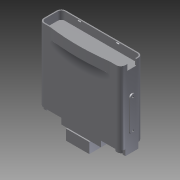
# Autodesk Inventor part: radio
Saved by Autodesk Inventor 2014 (Build 180170000, 170)
## iProperties
Created: 2013-11-09
Part Number: radio
Material: Generic
Document SubType Name: Modeling
Designer: Tyler
Density: 1 g/cm^3
Appearance: Default
Author: Tyler
Autodesk Inventor part; units mm, degrees
ref_plane "YZ Plane" through (0, 0, 0) normal (1, 0, 0) x (0, 1, 0)
ref_plane "XZ Plane" through (0, 0, 0) normal (0, 1, 0) x (-1, 0, 0)
ref_plane "XY Plane" through (0, 0, 0) normal (0, 0, 1) x (1, 0, 0)
sketch "Sketch1" plane through (0, 0, 0) normal (0, 0, 1) x (1, 0, 0)
  line L0 (-62, 19) -> (62, 19)
  line L1 (70, 11) -> (70, -11)
  line L2 (62, -19) -> (-62, -19)
  line L3 (-70, -11) -> (-70, 11)
  arc A0 (-62, 19) -> (-70, 11) centre (-62, 11) ccw
  arc A1 (-70, -11) -> (-62, -19) centre (-62, -11) ccw
  arc A2 (70, 11) -> (62, 19) centre (62, 11) ccw
  arc A3 (62, -19) -> (70, -11) centre (62, -11) ccw
  point P0 (0, 0)
  point P1 (70, -19)
  point P2 (70, 19)
  point P3 (-70, -19)
  dimension "d0" = 140
  dimension "d1" = 38
  dimension "d2" = 70
  dimension "d3" = 19
  dimension "d4" = 8
  dimension "d5" = 8
  dimension "d6" = 8
  dimension "d7" = 8
  constraints: 8 end point, 8 point on circle, 8 tangent, 6 point on line, 4 centre point, 2 parallel, 1 horizontal, 1 perpendicular
  measures "d0" distance of point (70, -19) point (-70, -19)
  measures "d1" distance of point (70, 19) point (70, -19)
  measures "d2" distance from line of L3 point (0, 0)
  measures "d3" distance from line of L2 point (0, 0)
  measures "d4" radius of A0
  measures "d5" radius of A1
  measures "d6" radius of A2
  measures "d7" radius of A3
extrude "Extrusion1" add sketch "Sketch1" against normal blind 18
sketch "Sketch2" plane through (0, 0, 0) normal (0, 0, 1) x (1, 0, 0)
  line L0 (-62, 19) -> (62, 19) projected
  arc A0 (-62, 19) -> (-70, 11) centre (-62, 11) ccw projected
  line L1 (-70, -11) -> (-70, 11) projected
  arc A1 (-70, -11) -> (-62, -19) centre (-62, -11) ccw projected
  line L2 (62, -19) -> (-62, -19) projected
  arc A2 (62, -19) -> (70, -11) centre (62, -11) ccw projected
  line L3 (70, 11) -> (70, -11) projected
  arc A3 (70, 11) -> (62, 19) centre (62, 11) ccw projected
  line L4 (62, 17) -> (-62, 17)
  arc A4 (-62, 17) -> (-68, 11) centre (-62, 11) ccw
  line L5 (-68, 11) -> (-68, -11)
  arc A5 (-68, -11) -> (-62, -17) centre (-62, -11) ccw
  line L6 (-62, -17) -> (62, -17)
  arc A6 (62, -17) -> (68, -11) centre (62, -11) ccw
  line L7 (68, -11) -> (68, 11)
  arc A7 (68, 11) -> (62, 17) centre (62, 11) ccw
  point P0 (0, 0)
  dimension "d10" = 2
  constraints: 8 end point, 8 point on circle, 4 centre point, 7 other
  measures "d10" distance between parallel lines of L4 L0
extrude "Extrusion2" cut sketch "Sketch2" against normal blind 14 contours A7 L7 A6 L6 A5 L5 A4 L4
sketch "Sketch3" plane through (70, -11, 0) normal (1, 0, 0) x (0, 0, -1)
  line L0 (0, 22) -> (0, 0) projected
  line L1 (-6.9158, 18.5) -> (10, 18.5)
  line L2 (10, 18.5) -> (10, 3.5)
  line L3 (10, 3.5) -> (-6.9158, 3.5)
  line L4 (-6.9158, 3.5) -> (-6.9158, 18.5)
  point P0 (0, 11)
  dimension "d13" = 6.9158
  dimension "d14" = 10
  dimension "d15" = 15
  dimension "d16" = 7.5
  constraints: 8 end point, 2 parallel, 1 horizontal, 1 perpendicular
  measures "d13" distance between parallel lines of L4 L0
  measures "d14" distance between parallel lines of L2 L0
  measures "d15" distance of L1.end L2.end
  measures "d16" distance from line of L3 point (0, 11)
extrude "Extrusion3" cut sketch "Sketch3" against normal blind 14
sketch "Sketch4" plane through (0, 0, -14) normal (0, 0, 1) x (1, 0, 0)
  line L0 (-62, -17) -> (62, -17) projected
  line L1 (62, 17) -> (-62, 17) projected
  line L2 (27, 19) -> (32, 19)
  line L3 (32, 19) -> (32, 16)
  line L4 (32, 16) -> (27, 16)
  line L5 (27, 16) -> (27, 19)
  line L6 (32, -19) -> (27, -19)
  line L7 (27, -19) -> (27, -16)
  line L8 (27, -16) -> (32, -16)
  line L9 (32, -16) -> (32, -19)
  line L10 (-42, -19) -> (-47, -19)
  line L11 (-47, -19) -> (-47, -16)
  line L12 (-47, -16) -> (-42, -16)
  line L13 (-42, -16) -> (-42, -19)
  line L14 (70, 7.5) -> (70, -7.5) projected
  line L15 (62, -19) -> (-62, -19) projected
  line L16 (-62, 19) -> (62, 19) projected
  line L17 (-39, 19) -> (-34, 19)
  line L18 (-34, 19) -> (-34, 16)
  line L19 (-34, 16) -> (-39, 16)
  line L20 (-39, 16) -> (-39, 19)
  line L21 (-70, -11) -> (-70, 11) projected
  point P0 (0, 0)
  dimension "d19" = 38
  dimension "d20" = 5
  dimension "d21" = 5
  dimension "d22" = 38
  dimension "d23" = 1
  dimension "d24" = 1
  dimension "d25" = 0
  dimension "d26" = 0
  dimension "d28" = 1
  dimension "d29" = 0
  dimension "d30" = 5
  dimension "d31" = 5
  dimension "d33" = 1
  dimension "d34" = 0
  dimension "d59" = 66
  dimension "d60" = 74
  constraints: 32 end point, 8 parallel, 4 horizontal, 4 perpendicular
  measures "d19" distance from line of L6.start L14
  measures "d20" distance between parallel lines of L9 L7
  measures "d21" distance between parallel lines of L5 L3
  measures "d22" distance between parallel lines of L14 L3
  measures "d23" distance between parallel lines of L4 L1
  measures "d24" distance between parallel lines of L0 L8
  measures "d25" distance between parallel lines of L15 L6
  measures "d26" distance between parallel lines of L16 L2
  measures "d28" distance between parallel lines of L19 L1
  measures "d29" distance between parallel lines of L16 L17
  measures "d30" distance of L18.end L19.end
  measures "d31" distance of L11.end L12.end
  measures "d33" distance between parallel lines of L0 L12
  measures "d34" distance between parallel lines of L15 L10
  measures "d59" distance of L3.end L18.end
  measures "d60" distance between parallel lines of L9 L13
extrude "Extrusion4" add sketch "Sketch4" along normal blind 13 contours L11 L12 L13 L0 | L0 L13 L10 L11 | L7 L8 L9 L0 | L0 L9 L6 L7 | L3 L4 L5 L1 | L1 L5 L2 L3 | L18 L19 L20 L1 | L1 L20 L16 L18
chamfer "Chamfer1" distance 1 distance2 1 1 edges at (-36.5, 16, -1) measured on face at (-36.5, 16, -1.5)
chamfer "Chamfer3" distance 1 distance2 1 1 edges at (29.5, 16, -1) measured on face at (29.5, 16, -1.5)
chamfer "Chamfer4" distance 1 distance2 1 1 edges at (-44.5, -16, -1) measured on face at (-44.5, -16, -1.5)
chamfer "Chamfer5" distance 1 distance2 1 1 edges at (29.5, -16, -1) measured on face at (29.5, -16, -1.5)
sketch "Sketch5" plane through (0, 0, -14) normal (0, 0, 1) x (1, 0, 0)
  line L0 (-39, 17) -> (-62, 17) projected
  arc A0 (-62, 17) -> (-68, 11) centre (-62, 11) ccw projected
  line L1 (-68, 11) -> (-68, -11) projected
  arc A1 (-68, -11) -> (-62, -17) centre (-62, -11) ccw projected
  line L2 (-62, -17) -> (-47, -17) projected
  line L3 (-47, -17) -> (-47, -16) projected
  line L4 (-47, -16) -> (-42, -16) projected
  line L5 (-42, -16) -> (-42, -17) projected
  line L6 (-42, -17) -> (27, -17) projected
  line L7 (27, -17) -> (27, -16) projected
  line L8 (27, -16) -> (32, -16) projected
  line L9 (32, -16) -> (32, -17) projected
  line L10 (32, -17) -> (62, -17) projected
  line L11 (-49, 17) -> (37, 17)
  line L12 (37, 17) -> (37, -17)
  line L13 (37, -17) -> (-49, -17)
  line L14 (-49, -17) -> (-49, 17)
  point P0 (32, 16)
  point P1 (-39, 16)
  point P2 (0, 0)
  dimension "d53" = 10
  dimension "d54" = 5
  constraints: 8 end point, 2 parallel, 2 point on line, 1 horizontal, 1 perpendicular
  measures "d53" distance from line of point (-39, 16) L14
  measures "d54" distance from line of point (32, 16) L12
extrude "Extrusion5" cut sketch "Sketch5" along normal blind 11
sketch "Sketch8" plane through (0, 0, 0) normal (0, 0, 1) x (1, 0, 0)
  line L0 (-70, -11) -> (-70, 11) projected
  line L1 (62, -19) -> (-62, -19) projected
  line L2 (70, -7.5) -> (70, -11) projected
  line L3 (62, -17) -> (-62, -17) projected
  line L4 (0, -22.5) -> (0, -17) construction
  arc A0 (-52, -18.8579) -> (52, -18.8579) centre (0, 350.5357) ccw
  arc A1 (-49.9899, -19.1353) -> (-52, -19) centre (-52, -34) ccw
  arc A2 (52, -19) -> (49.9899, -19.1353) centre (52, -34) ccw
  line L5 (-52, -19) -> (-52, -17)
  line L6 (52, -19) -> (52, -17)
  line L7 (52, -17) -> (-52, -17)
  point P0 (0, 0)
  dimension "d63" = 2
  dimension "d64" = 18
  dimension "d65" = 18
  dimension "d66" = 5.5
  dimension "d67" = 30
  dimension "d68" = 30
  constraints: 9 point on circle, 8 end point, 6 point on line, 4 tangent, 3 centre point, 3 perpendicular, 1 collinear, 1 midpoint
  measures "d63" distance between parallel lines of L1 L3
  measures "d64" distance from line of L2 A2.centre
  measures "d65" distance from line of A1.centre L0
  measures "d66" distance of L4.start L4.end
  measures "d67" diameter of A1
  measures "d68" diameter of A2
extrude "Extrusion8" add sketch "Sketch8" against normal up to surface (18 mm away) contours A0 L1 | L1 A0 L5 L3 L6
sketch "Sketch11" plane through (0, 0, -18) normal (0, 0, -1) x (-1, 0, 0)
  line L0 (62, -19) -> (50.9804, -19) projected
  arc A0 (62, -19) -> (70, -11) centre (62, -11) ccw projected
  line L1 (70, 11) -> (70, -11) projected
  arc A1 (70, 11) -> (62, 19) centre (62, 11) ccw projected
  line L2 (-62, 19) -> (62, 19) projected
  arc A2 (-62, 19) -> (-70, 11) centre (-62, 11) ccw projected
  line L3 (-70, -11) -> (-70, 11) projected
  arc A3 (-70, -11) -> (-62, -19) centre (-62, -11) ccw projected
  line L4 (-50.9804, -19) -> (-62, -19) projected
  line L5 (-50.9804, -19) -> (50.9804, -19)
  point P0 (0, 0)
  constraints: 2 end point, 1 collinear
extrude "Extrusion10" add sketch "Sketch11" along normal blind 107
fillet "Fillet2" radius 60 1 edges at (0, -19, -18)
sketch "Sketch12" plane through (0, 0, -125) normal (0, 0, -1) x (-1, 0, 0)
  line L0 (-62, -19) -> (62, -19) projected
  line L1 (-70, 11) -> (-70, -11) projected
  circle A0 centre (-50, 2) radius 7.5
  point P0 (0, 0)
  dimension "d81" = 15
  dimension "d82" = 21
  dimension "d83" = 20
  constraints: 1 centre point
  measures "d81" diameter of A0
  measures "d82" distance from line of L0 A0.centre
  measures "d83" distance from line of L1 A0.centre
extrude "Extrusion11" add sketch "Sketch12" along normal blind 17
sketch "Sketch13" plane through (0, 0, -125) normal (0, 0, -1) x (-1, 0, 0)
  line L0 (70, -11) -> (70, 11) projected
  line L1 (-70, 11) -> (-70, -11) projected
  line L2 (-70, 11) -> (-65, 11)
  line L3 (-65, 11) -> (-65, -11)
  line L4 (-65, -11) -> (-70, -11)
  line L5 (-70, -11) -> (-70, 11)
  line L6 (70, -11) -> (65, -11)
  line L7 (65, -11) -> (65, 11)
  line L8 (65, 11) -> (70, 11)
  line L9 (70, 11) -> (70, -11)
  point P0 (0, 0)
  dimension "d86" = 0
  dimension "d87" = 0
  dimension "d88" = 0
  dimension "d89" = 5
  dimension "d90" = 0
  dimension "d91" = 0
  dimension "d92" = 0
  dimension "d93" = 5
  constraints: 16 end point, 4 parallel, 2 horizontal, 2 perpendicular
  measures "d86" distance from line of L2 L1.start
  measures "d87" distance from line of L1.end L4
  measures "d88" distance between parallel lines of L1 L5
  measures "d89" distance between parallel lines of L1 L3
  measures "d90" distance between parallel lines of L0 L9
  measures "d91" distance from line of L8 L0.end
  measures "d92" distance from line of L0.start L6
  measures "d93" distance between parallel lines of L9 L7
extrude "Extrusion12" add sketch "Sketch13" along normal blind 10
sketch "Sketch14" plane through (0, 0, -125) normal (0, 0, -1) x (-1, 0, 0)
  line L0 (-62, -19) -> (62, -19) projected
  line L1 (62, 19) -> (-62, 19) projected
  line L2 (-36, 19) -> (32, 19)
  line L3 (32, 19) -> (32, -19)
  line L4 (32, -19) -> (-36, -19)
  line L5 (-36, -19) -> (-36, 19)
  line L6 (70, -11) -> (70, 11) projected
  point P0 (0, 0)
  dimension "d96" = 38
  dimension "d97" = 68
  dimension "d98" = 0
  dimension "d99" = 0
  constraints: 8 end point, 2 parallel, 1 horizontal, 1 perpendicular
  measures "d96" distance between parallel lines of L3 L6
  measures "d97" distance of L2.start L2.end
  measures "d98" distance between parallel lines of L0 L4
  measures "d99" distance between parallel lines of L1 L2
extrude "Extrusion13" add sketch "Sketch14" along normal blind 10
sketch "Sketch15" plane through (0, 0, -135) normal (0, 0, -1) x (-1, 0, 0)
  line L0 (32, 19) -> (-36, 19) projected
  line L1 (32, -19) -> (32, 19) projected
  line L2 (-18, 19) -> (22, 19)
  line L3 (22, 19) -> (22, -21)
  line L4 (22, -21) -> (-18, -21)
  line L5 (-18, -21) -> (-18, 19)
  point P0 (0, 0)
  dimension "d102" = 40
  dimension "d103" = 40
  dimension "d104" = 0
  dimension "d105" = 10
  constraints: 8 end point, 2 parallel, 1 horizontal, 1 perpendicular
  measures "d102" distance of L2.start L2.end
  measures "d103" distance of L4.end L2.start
  measures "d104" distance between parallel lines of L0 L2
  measures "d105" distance between parallel lines of L1 L3
extrude "Extrusion14" add sketch "Sketch15" along normal blind 18
sketch "Sketch16" plane through (70, -11, 0) normal (1, 0, 0) x (0, 0, -1)
  arc A0 (52, 16) -> (52, 6) centre (52, 11) ccw
  arc A1 (102, 6) -> (102, 16) centre (102, 11) ccw
  line L0 (0, 0) -> (0, 22) projected
  line L1 (52, 16) -> (102, 16)
  line L2 (102, 6) -> (52, 6)
  line L3 (0, 30) -> (125, 30) projected
  line L4 (0, -8) -> (125, -8) projected
  point P0 (0, 11)
  dimension "d108" = 52
  dimension "d109" = 10
  dimension "d110" = 10
  dimension "d111" = 50
  dimension "d113" = 19
  dimension "d114" = 19
  constraints: 4 end point, 4 point on circle, 4 tangent, 2 centre point, 1 perpendicular
  measures "d108" distance from line of L0 A0.centre
  measures "d109" diameter of A0
  measures "d110" diameter of A1
  measures "d111" distance of A0.centre A1.centre
  measures "d113" distance from line of L3 A0.centre
  measures "d114" distance from line of L4 A0.centre
extrude "Extrusion15" add sketch "Sketch16" along normal blind 2 and the other way blind 142
hole "Hole1" at (72, 0, -102) direction (-1, 0, 0) diameter 3.242 depth 8 tip angle 118 thread size "M4x0.7" designation "M4" class "6H" standard "GB Metric profile"
hole "Hole2" at (72, 0, -52) direction (-1, 0, 0) diameter 3.242 depth 8 tip angle 118 thread size "M4x0.7" designation "M4" class "6H" standard "GB Metric profile"
hole "Hole3" at (-72, 0, -52) direction (1, 0, 0) diameter 3.242 depth 8 tip angle 118 thread size "M4x0.7" designation "M4" class "6H" standard "GB Metric profile"
hole "Hole4" at (-72, 0, -102) direction (1, 0, 0) diameter 3.242 depth 8 tip angle 118 thread size "M4x0.7" designation "M4" class "6H" standard "GB Metric profile"
equation "\"d2\" = 0.5 * d0"
equation "\"d3\" = 0.5 * d1"
equation "\"d16\" = 0.5 * d15"
equation "\"d114\" = d113"
body "Solid1"
